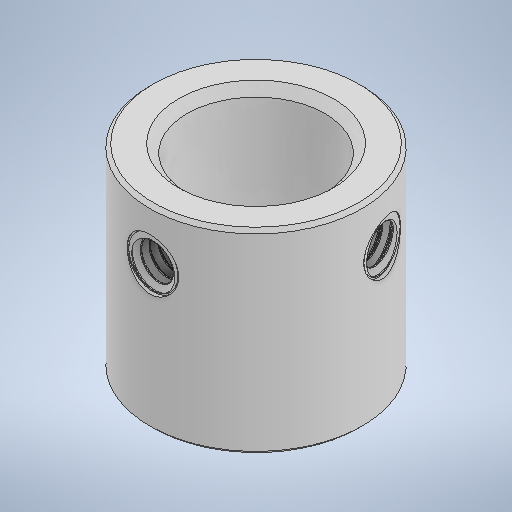
# Autodesk Inventor part: Collar 8x12.35x11.35
Saved by Autodesk Inventor 2025.2 (Build 292293000, 293)
## iProperties
Created: 2021-04-20
Part Number: Collar 8x12.35x11.35
Material: Generic
Document SubType Name: Modeling
Designer: Johnson Ebenezer R
Density: 1 g/cm^3
Appearance: Default
Author: Johnson Ebenezer R
Autodesk Inventor part; units mm, degrees
ref_plane "YZ Plane" through (0, 0, 0) normal (1, 0, 0) x (0, 1, 0)
ref_plane "XZ Plane" through (0, 0, 0) normal (0, 1, 0) x (-1, 0, 0)
sketch "Sketch1" plane through (0, 0, 0) normal (0, 1, 0) x (-1, 0, 0)
  circle A0 centre (0, 0) radius 6.175
  circle A1 centre (0, 0) radius 4
  dimension "d8" = 8
  dimension "d9" = 12.35
  constraints: 2 centre point, 2 coincident
  measures "d8" diameter of A1
  measures "d9" diameter of A0
extrude "Extrusion1" add sketch "Sketch1" along normal blind 11.35
chamfer "Chamfer1" distance 0.5 angle 45 2 edges at (4, 0, 0) (4, 11.35, 0)
chamfer "Chamfer2" distance 0.2 angle 45 2 edges at (6.175, 11.35, 0) (6.175, 0, 0)
ref_plane "Work Plane1" through (0, 0, 6.175) normal (0, 0, 1) x (1, 0, 0)
sketch "Sketch2" plane through (0, 0, 6.175) normal (0, 0, 1) x (1, 0, 0)
  line L0 (4.5, 11.35) -> (-4.5, 11.35) projected
  line L1 (0, 11.35) -> (0, 8.35) construction
  point P0 (0, 0)
  dimension "d11" = 3
  constraints: 2 end point, 1 midpoint, 1 vertical
  measures "d11" distance of L1.start L1.end
hole "Hole1" at (0, 8.35, 6.175) direction (0, 0, -1) diameter 2.85 depth 6.175 counterbore diameter 3 counterbore depth 0.2
thread "Thread1" size "M3x0.5" class "6H" standard "ANSI Metric M Profile" length 2
sketch "Sketch4" plane through (0, 8.35, 5.975) normal (-1, 0, 0) x (0, 1, 0)
  line L0 (1.425, 0) -> (1.425, 2)
  line L1 (1.425, 2) -> (1.0543, 2)
  line L2 (1.0543, 2) -> (1.0543, 0)
  line L3 (1.0543, 0) -> (1.425, 0)
  line L4 (0, -3.0844) -> (0, 14.6891) projected
  constraints: 8 end point
revolve "Revolution1" add sketch "Sketch4" angle 360 about axis through (0, 8.35, 5.975) along (0, 0, -1) separate body
sketch "Sketch3" plane through (0, 9.775, 5.975) normal (1, 0, 0) x (0, 0, -1)
  line L0 (-0.2918, -0.0255) -> (-0.2501, -0.0255) construction
  line L1 (0.0416, -0.3456) -> (-0.0001, -0.4257) construction
  line L2 (-0.5001, -0.4257) -> (-0.5418, -0.3456) construction
  line L3 (-0.2084, -0.0255) -> (-0.2501, 0.0546) construction
  line L4 (-0.2501, 0.0546) -> (-0.2918, -0.0255) construction
  line L5 (-0.5001, -0.4257) -> (-0.4584, -0.3456) construction
  line L6 (-0.2084, -0.0255) -> (-0.0418, -0.3456)
  line L7 (-0.5418, -0.3456) -> (-0.4584, -0.3456) construction
  arc A0 (-0.5418, -0.3456) -> (-0.5001, -0.3709) centre (-0.5001, -0.3239) ccw construction
  line L8 (0.0416, -0.3456) -> (-0.0418, -0.3456) construction
  line L9 (-0.5001, -0.4257) -> (-0.5001, -0.3456) construction
  line L10 (-0.0001, -0.4257) -> (-0.0001, -0.3456) construction
  line L11 (-0.2501, 0.0546) -> (-0.2501, -0.0002) construction
  line L12 (-0.5001, -0.3709) -> (-0.0001, -0.3709)
  arc A1 (-0.5001, -0.3709) -> (-0.4584, -0.3456) centre (-0.5001, -0.3239) ccw
  line L13 (-0.0418, -0.3456) -> (-0.0001, -0.4257) construction
  line L14 (-0.4584, -0.3456) -> (-0.2918, -0.0255)
  line L15 (-0.0001, -0.0002) -> (-0.0001, 0.0177)
  line L16 (-0.0001, 0.0177) -> (-0.0001, -0.0002)
  line L17 (-0.0001, -0.0002) -> (0.0334, -0.0002)
  arc A2 (-0.0418, -0.3456) -> (-0.0001, -0.3709) centre (-0.0001, -0.3239) ccw
  arc A3 (-0.0001, -0.3709) -> (0.0416, -0.3456) centre (-0.0001, -0.3239) ccw construction
  arc A4 (-0.2501, -0.0002) -> (-0.2918, -0.0255) centre (-0.2501, -0.0471) ccw
  arc A5 (-0.2084, -0.0255) -> (-0.2501, -0.0002) centre (-0.2501, -0.0471) ccw
  line L18 (-0.2501, -0.0002) -> (-0.2501, -0.0255) construction
  line L19 (-0.2501, -0.0255) -> (-0.2084, -0.0255) construction
  dimension "d21" = 55
  dimension "d22" = 0.08
  dimension "d23" = 0.08
  dimension "Sketch3_ThreadOffset" = 0
  dimension "Sketch3_MajorRadius" = 0.3707
  dimension "d26" = 0.5
  dimension "Sketch3_MinorRadius" = 0
  constraints: 40 end point, 12 point on circle, 10 parallel, 8 tangent, 6 centre point, 6 collinear, 2 midpoint, 2 point on line, 1 horizontal, 1 perpendicular, 3 other
  measures "d21" angle of L6 L14
  measures "d22" distance of L3.end L0.end
  measures "d23" distance of L1.end L10.end
  measures "Sketch3_ThreadOffset" distance between parallel lines of L15 L10
  measures "Sketch3_MajorRadius" distance from line of L12 L15.start
  measures "d26" distance from line of L1.end L9
  measures "Sketch3_MinorRadius" distance edge to line of A5 L17
coil "Coil1" sketch "Sketch3" operation cut axis through (0, 8.35, 5.975) along (0, 0, -1) pitch 0.5005 turns 5.994006 hand right bodies 2
pattern_circular "Circular Pattern1" count 2 over 105 about axis through (0, 0, 0) along (0, 1, 0) of "Hole1", "Revolution1", "Coil1" bodies 1
equation "\"d17\" = 0.5 * d9"
equation "\"d21\" = d28"
equation "\"d22\" = 0.160083 * Sketch3_Pitch"
equation "\"d23\" = 0.160083 * Sketch3_Pitch"
equation "\"d26\" = Sketch3_Pitch"
equation "\"d10\" = 0.5 * d9"
equation "\"d28\" = 55deg"
equation "\"Sketch3_Pitch\" = 0.5"
body "Solid1"
body "Solid2"
